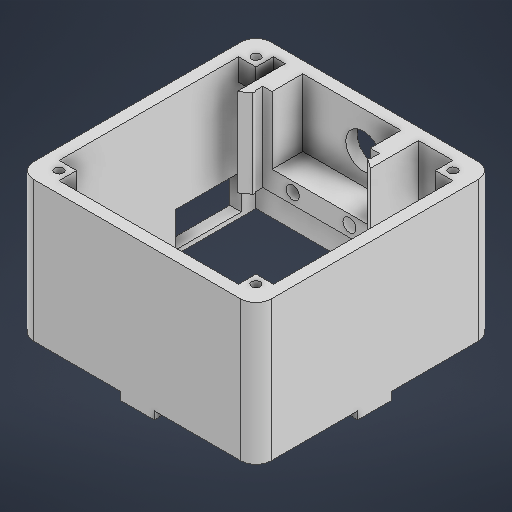
# Autodesk Inventor part: brick_shell_+USB_nudge_V3
Saved by Autodesk Inventor 2026.2 (Build 302298010, 298A)
## iProperties
Created: 2026-03-17
Part Number: brick_shell_+USB_nudge_V3
Material: Generisch
Document SubType Name: Modeling
Designer: ami-student
Density: 1 g/cm^3
Appearance: Vorgabe
Author: ami-student
Autodesk Inventor part; units mm, degrees
ref_plane "YZ Plane" through (0, 0, 0) normal (1, 0, 0) x (0, 1, 0)
ref_plane "XZ Plane" through (0, 0, 0) normal (0, 1, 0) x (-1, 0, 0)
sketch "Skizze1" plane through (0, 0, 0) normal (0, 0, 1) x (1, 0, 0)
  line L0 (-27.13, -27.13) -> (27.13, -27.13)
  line L1 (27.13, -27.13) -> (27.13, 27.13)
  line L2 (27.13, 27.13) -> (-27.13, 27.13)
  line L3 (-27.13, 27.13) -> (-27.13, -27.13)
  line L4 (-37.982, 0) -> (37.982, 0) construction
  line L5 (0, -37.982) -> (0, 37.982) construction
  line L6 (-24.484, 24.484) -> (24.484, 24.484)
  line L7 (24.484, 24.484) -> (24.484, -24.484)
  line L8 (24.484, -24.484) -> (-24.484, -24.484)
  line L9 (-24.484, -24.484) -> (-24.484, 24.484)
  point P0 (0, 0)
  dimension "d0" = 54.26
  dimension "d1" = 2.646
  constraints: 16 end point, 4 parallel, 4 perpendicular, 2 horizontal, 4 other
  measures "d0" distance between parallel lines of L1 L3
  measures "d1" distance between parallel lines of L9 L3
extrude "Extrusion1" add sketch "Skizze1" along normal blind 32
fillet "Rundung1" radius 3.5 4 edges at (-27.13, 27.13, 16) (27.13, 27.13, 16) (-27.13, -27.13, 16) (27.13, -27.13, 16)
sketch "Skizze2" plane through (0, 0, 32) normal (0, 0, 1) x (1, 0, 0)
  line L0 (-24.484, -24.484) -> (-24.484, 24.484) projected
  line L1 (-24.484, 24.484) -> (24.484, 24.484) projected
  line L2 (-24.484, 20.484) -> (-20.484, 20.484)
  line L3 (-20.484, 20.484) -> (-20.484, 24.484)
  line L4 (-20.484, 24.484) -> (-24.484, 24.484)
  line L5 (-24.484, 24.484) -> (-24.484, 20.484)
  point P0 (0, 0)
  point P1 (-24.484, 20.984)
  point P2 (-20.984, 24.484)
  point P3 (20.984, 24.484)
  point P4 (-24.484, 20.984)
  point P5 (-20.984, 24.484)
  dimension "d5" = 4
  constraints: 8 end point, 2 parallel, 2 perpendicular, 2 point on line, 1 horizontal
  measures "d5" distance of L2.end L3.end
extrude "Extrusion2" add sketch "Skizze2" against normal blind 5
sketch "Skizze3" plane through (0, 0, 32) normal (0, 0, 1) x (1, 0, 0)
  line L0 (-24.484, 20.484) -> (-20.484, 20.484) projected
  line L1 (-20.484, 20.484) -> (-20.484, 24.484) projected
  point P0 (0, 0)
  point P1 (-22.484, 22.484)
  dimension "d8" = 2
  dimension "d9" = 2
  measures "d8" distance from line of L0 point (-22.484, 22.484)
  measures "d9" distance from line of L1 point (-22.484, 22.484)
hole "Bohrung1" at (-22.484, 22.484, 32) direction (0, 0, -1) diameter 2 depth 5
pattern_circular "Runde Anordnung1" count 4 over 360 about axis through (0, 0, -10) along (0, 0, 1) of "Extrusion2", "Bohrung1"
sketch "Skizze4" plane through (-20.984, 24.484, 0) normal (0, -1, 0) x (1, 0, 0)
  line L0 (41.468, 27) -> (41.468, 32) projected
  line L1 (0.5, 32) -> (41.468, 32) projected
  line L2 (0.5, 32) -> (0.5, 27) projected
  line L3 (0.5, 27) -> (-3.5, 27) projected
  line L4 (-3.5, 0) -> (45.468, 0) projected
  line L5 (45.468, 27) -> (41.468, 27) projected
  line L6 (44.614, 32) -> (-2.646, 32) projected
  line L7 (3.184, 32) -> (7.184, 32)
  line L8 (7.184, 32) -> (7.184, 11.949)
  line L9 (7.184, 11.949) -> (3.184, 11.949)
  line L10 (3.184, 11.949) -> (3.184, 32)
  line L11 (7.184, 11.949) -> (29.6, 11.949)
  line L12 (29.6, 11.949) -> (29.6, 16.63)
  line L13 (29.6, 16.63) -> (7.184, 16.63)
  line L14 (7.184, 16.63) -> (7.184, 11.949)
  line L15 (0.5, 32) -> (41.468, 32) projected
  line L16 (29.6, 11.949) -> (33.6, 11.949)
  line L17 (33.6, 11.949) -> (33.6, 32)
  line L18 (33.6, 32) -> (29.6, 32)
  line L19 (29.6, 32) -> (29.6, 11.949)
  line L20 (-3.5, 0) -> (-3.5, 27) projected
  line L21 (45.468, 0) -> (45.468, 27) projected
  point P0 (20.984, 0)
  point P1 (18.392, 11.949)
  point P2 (33.6, 32)
  point P3 (7.184, 16.63)
  dimension "d20" = 4
  dimension "d21" = 4.681
  dimension "d22" = 22.416
  dimension "d23" = 2.684
  dimension "d24" = 15.37
  constraints: 24 end point, 6 parallel, 3 horizontal, 3 perpendicular, 2 point on line, 1 collinear, 1 midpoint
  measures "d20" distance between parallel lines of L8 L10
  measures "d21" distance from line of L13 point (18.392, 11.949)
  measures "d22" distance between parallel lines of L19 L8
  measures "d23" distance between parallel lines of L10 L2
  measures "d24" distance between parallel lines of L1 L13
extrude "Extrusion3" add sketch "Skizze4" along normal blind 7.023 contours L17 L16 L12 L19 L1 | L8 L9 L10 L1 | L12 L11 L8 L13
sketch "Skizze5" plane through (0, 0, 32) normal (0, 0, 1) x (1, 0, 0)
  line L0 (-17.8, 17.461) -> (12.616, 17.461) projected
  line L1 (-17.8, 17.461) -> (-15.9, 17.461)
  line L2 (-17.8, 15.0145) -> (-17.8, 17.461)
  line L3 (-17.8, 15.0145) -> (-17.8, 13.484)
  line L4 (-17.8, 13.484) -> (-15.806, 14.94)
  line L5 (-20.484, 24.484) -> (-17.8, 24.484) projected
  arc A0 (-15.806, 14.94) -> (-15.9, 15.637) centre (-16.0419, 15.263) ccw
  line L6 (-15.9, 15.637) -> (-15.9, 17.461)
  point P0 (0, 0)
  dimension "d27" = 11
  dimension "d30" = 0.4
  dimension "d31" = 1.824
  dimension "d32" = 1.9
  dimension "d33" = 1.994
  constraints: 10 end point, 2 point on circle, 2 vertical, 1 centre point, 1 horizontal, 1 tangent
  measures "d27" distance from line of L5 L3.end
  measures "d30" radius of A0
  measures "d31" distance of L1.end L6.start
  measures "d32" distance between parallel lines of L6 L2
  measures "d33" horizontal distance of L3.end L4.end
extrude "Extrusion4" add sketch "Skizze5" against normal up to surface (20.051 mm away)
ref_plane "Arbeitsebene1" through (-2.592, 17.461, 16.63) normal (1, 0, 0) x (0, 0, -1)
sketch "Skizze7" plane through (-20.984, 17.461, 0) normal (0, -1, 0) x (1, 0, 0)
  line L0 (33.6, 32) -> (29.6, 32) projected
  line L1 (29.6, 32) -> (29.6, 16.63) projected
  line L2 (29.6, 16.63) -> (7.184, 16.63) projected
  line L3 (7.184, 16.63) -> (7.184, 32) projected
  line L4 (7.184, 32) -> (5.084, 32) projected
  line L5 (5.084, 32) -> (5.084, 11.949) projected
  line L6 (5.084, 11.949) -> (33.6, 11.949) projected
  line L7 (33.6, 11.949) -> (33.6, 32) projected
  point P0 (20.984, 0)
  point P1 (11.915, 14.413)
  dimension "d36" = 2.464
  dimension "d37" = 4.731
  measures "d36" distance from line of point (11.915, 14.413) L6
  measures "d37" distance from line of L3 point (11.915, 14.413)
hole "Bohrung2" at (-9.069, 17.461, 14.413) direction (0, 1, 0) diameter 3 depth 7.023
mirror "Spiegeln2" about plane through (-2.592, 17.461, 16.63) normal (1, 0, 0) of "Extrusion4", "Bohrung2"
sketch "Skizze8" plane through (-23.63, 27.13, 0) normal (0, 1, 0) x (1, 0, 0)
  line L0 (47.26, -32) -> (0, -32) projected
  line L1 (23.63, -32) -> (23.63, 0) construction
  point P0 (23.63, -23.607)
  dimension "d45" = 8.393
  constraints: 2 end point, 1 midpoint, 1 point on line, 1 vertical
  measures "d45" distance from line of L0 point (23.63, -23.607)
hole "Bohrung3" at (0, 27.13, 23.607) direction (0, -1, 0) diameter 8 depth 2.646
sketch "Skizze9" plane through (0, 0, 0) normal (0, 0, -1) x (-1, 0, 0)
  line L0 (-23.63, 27.13) -> (23.63, 27.13) projected
  line L1 (13.8, 24.484) -> (-8.616, 24.484) projected
  line L2 (-3.9, 27.13) -> (3.9, 27.13)
  line L3 (3.9, 27.13) -> (3.9, 24.484)
  line L4 (3.9, 24.484) -> (-3.9, 24.484)
  line L5 (-3.9, 24.484) -> (-3.9, 27.13)
  line L6 (0, -37.982) -> (0, 37.982) construction
  point P0 (0, 0)
  dimension "d53" = 7.8
  constraints: 8 end point, 2 parallel, 2 point on line, 1 horizontal, 1 perpendicular, 1 other
  measures "d53" distance between parallel lines of L3 L5
extrude "Extrusion5" add sketch "Skizze9" along normal blind 1.8
pattern_circular "Runde Anordnung2" count 4 over 360 about axis through (0, 0, -10) along (0, 0, 1) of "Extrusion5"
sketch "Skizze10" plane through (-27.13, -23.63, 32) normal (-1, 0, 0) x (0, 0, 1)
  line L0 (-23, 44.76) -> (-31, 44.76)
  line L1 (-31, 44.76) -> (-31, 29.76)
  line L2 (-31, 29.76) -> (-23, 29.76)
  line L3 (-23, 29.76) -> (-23, 44.76)
  line L4 (0, 50.76) -> (-32, 50.76) projected
  line L5 (-32, 47.26) -> (-32, 27.53) projected
  point P0 (-32, 23.63)
  dimension "d59" = 6
  dimension "d60" = 8
  dimension "d61" = 15
  dimension "d62" = 1
  constraints: 8 end point, 2 parallel, 1 horizontal, 1 perpendicular
  measures "d59" distance between parallel lines of L4 L0
  measures "d60" distance between parallel lines of L3 L1
  measures "d61" distance of L2.end L0.start
  measures "d62" distance between parallel lines of L5 L1
extrude "Extrusion6" cut sketch "Skizze10" against normal up to surface (2.646 mm away)
